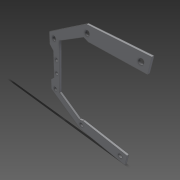
# Autodesk Inventor part: MuzzleHeadMount
Saved by Autodesk Inventor 2020 (Build 240168000, 168)
## iProperties
Created: 2021-07-18
Part Number: MuzzleHeadMount
Material: Generic
Document SubType Name: Sheet Metal
Designer: valer
Density: 1 g/cm^3
Sheet Metal Rule: Default
Appearance: Default
Author: valer
Autodesk Inventor part; units mm, degrees
ref_plane "YZ Plane" through (0, 0, 0) normal (1, 0, 0) x (0, 1, 0)
ref_plane "XZ Plane" through (0, 0, 0) normal (0, 1, 0) x (-1, 0, 0)
ref_plane "XY Plane" through (0, 0, 0) normal (0, 0, 1) x (1, 0, 0)
sketch "Sketch1" plane through (0, 0, 0) normal (0, 0, 1) x (1, 0, 0)
  circle A0 centre (0, 0) radius 3
  circle A1 centre (-6.2839, -68.2915) radius 2.875
  circle A2 centre (39.1052, -97.9753) radius 3
  circle A3 centre (99.0811, -103.4941) radius 3
  circle A4 centre (110.0198, 15.3837) radius 3
  circle A5 centre (50.0439, 20.9025) radius 3
  line L0 (-14.6913, -72.3521) -> (36.3914, -105.7594)
  line L1 (36.3914, -105.7594) -> (106.3144, -112.1934)
  line L2 (106.3144, -112.1934) -> (107.7805, -96.2608)
  line L3 (107.7805, -96.2608) -> (41.8191, -90.1913)
  line L4 (41.8191, -90.1913) -> (2.1235, -64.2309)
  line L5 (2.1235, -64.2309) -> (4.8244, -34.8788)
  line L6 (-178.2222, -18.0356) -> (255.5293, -57.9477) construction
  line L7 (-6.2839, -68.2915) -> (-3.142, -34.1457) construction
  line L8 (-6.2839, -68.2915) -> (39.1052, -97.9753) construction
  line L9 (39.1052, -97.9753) -> (99.0811, -103.4941) construction
  line L10 (-14.6913, -72.3521) -> (-11.1083, -33.4127)
  line L11 (4.8244, -34.8788) -> (-11.1083, -33.4127)
  line L12 (-7.5253, 5.5266) -> (48.7961, 29.0511)
  line L13 (48.7961, 29.0511) -> (118.7191, 22.617)
  line L14 (118.7191, 22.617) -> (117.2531, 6.6843)
  line L15 (117.2531, 6.6843) -> (51.2917, 12.7538)
  line L16 (51.2917, 12.7538) -> (7.5253, -5.5266)
  line L17 (7.5253, -5.5266) -> (4.8244, -34.8788)
  line L18 (-7.5253, 5.5266) -> (-11.1083, -33.4127)
  point P0 (0, 0)
  dimension "d0" = 8
  dimension "d1" = 8
  dimension "d2" = 8
  dimension "d3" = 8
  dimension "d4" = 8
  dimension "d5" = 8
  dimension "d6" = 8
  measures "d0" distance between parallel lines of L1 L9
  measures "d1" distance between parallel lines of L3 L9
  measures "d2" distance from line of L2 L9.end
  measures "d3" distance between parallel lines of L0 L8
  measures "d4" distance between parallel lines of L4 L8
  measures "d5" distance between parallel lines of L10 L7
  measures "d6" distance between parallel lines of L5 L7
extrude "Plate1" add sketch "Sketch1" along normal blind 3.048
sketch "Sketch2" plane through (0, 0, 3.048) normal (0, 0, 1) x (1, 0, 0)
  line L0 (-13.3312, -57.5708) -> (-6.8067, -52.1458)
  line L1 (-14.6913, -72.3521) -> (-7.5253, 5.5266) projected
  line L2 (7.5253, -5.5266) -> (2.1235, -64.2309) projected
  line L3 (-11.1083, -33.4127) -> (4.8244, -34.8788)
  line L4 (2.1235, -64.2309) -> (7.5253, -5.5266) projected
  line L5 (-6.8067, -52.1458) -> (-3.4604, -15.7791)
  line L6 (-3.4604, -15.7791) -> (-8.8854, -9.2546)
  point P0 (0, 0)
  point P1 (-5.1335, -33.9625)
  dimension "d8" = 45
  dimension "d9" = 45
  dimension "d10" = 6
  constraints: 8 end point, 3 midpoint, 3 point on line, 1 perpendicular
  measures "d8" angle of L1 L0
  measures "d9" angle of L1 L6
  measures "d10" distance between parallel lines of L1 L5
extrude "Cut1" cut sketch "Sketch2" against normal blind 3.048
sketch "Sketch3" plane through (0, 0, 3.048) normal (0, 0, 1) x (1, 0, 0)
  ellipse E0 centre (35.8905, -88.6417) end of major axis (36.1653, -85.6543) minor radius 2.9795 (33.3641, -87.0543) -> (38.664, -87.542) ccw projected
  ellipse E1 centre (45.1798, 12.3117) end of major axis (44.9049, 9.3243) minor radius 2.9795 (42.6535, 13.8991) -> (47.9534, 13.4114) ccw projected
  line L0 (41.8191, -90.1913) -> (107.7805, -96.2608) projected
  line L1 (41.8191, -90.1913) -> (35.3649, -91.8772)
  line L2 (35.3649, -91.8772) -> (1.6108, -69.8026)
  line L3 (7.5253, -5.5266) -> (2.1235, -64.2309) projected
  line L4 (1.6108, -69.8026) -> (2.1235, -64.2309)
  line L5 (2.1235, -64.2309) -> (41.8191, -90.1913) construction
  line L6 (-178.2222, -18.0356) -> (255.5293, -57.9477)
  line L7 (41.8191, -90.1913) -> (2.1235, -64.2309)
  line L8 (51.2917, 12.7538) -> (45.2535, 15.5893)
  line L9 (45.2535, 15.5893) -> (8.0379, 0.045)
  line L10 (8.0379, 0.045) -> (7.5253, -5.5266)
  line L11 (7.5253, -5.5266) -> (51.2917, 12.7538)
  point P0 (0, 0)
  constraints: 18 end point, 3 symmetric about line, 1 collinear, 1 parallel, 7 other
extrude "Cut2" cut sketch "Sketch3" against normal blind 3.048 contours L2 L4 L7 E0 | E0 L1 L2 | E0 L7 L1 | L11 L10 L9 L8
sketch "Sketch4" plane through (0, 0, 3.048) normal (0, 0, 1) x (1, 0, 0)
  line L0 (-3.4604, -15.7791) -> (-6.8067, -52.1458) projected
  line L1 (1.6108, -69.8026) -> (8.0379, 0.045) projected
  line L2 (-5.1335, -33.9625) -> (4.8244, -34.8788) construction
  line L3 (-0.1546, -34.4206) -> (-1.8277, -52.604) construction
  line L4 (-6.8067, -52.1458) -> (-3.4604, -15.7791) projected
  line L5 (-6.8067, -52.1458) -> (3.1512, -53.0621) construction
  circle A0 centre (-0.9912, -43.5123) radius 2.5
  circle A1 centre (0.682, -25.329) radius 2.5
  point P0 (0, 0)
  dimension "d15" = 5
  constraints: 6 end point, 5 midpoint, 2 centre point, 1 perpendicular, 1 point on line, 1 symmetric about line, 1 other
  measures "d15" diameter of A0
hole "Hole1" at (-0.9912, -43.5123, 3.048) at (0.682, -25.329, 3.048) direction (0, 0, -1) diameter 5 depth 3.048 tip angle 118
equation "\"d1\" = d0"
equation "\"d2\" = d0"
equation "\"d3\" = d0"
equation "\"d4\" = d0"
equation "\"d9\" = d8"
equation "\"d11\" = Thickness"
equation "\"d13\" = Thickness"
equation "\"d21\" = Thickness"
equation "\"d7\" = Thickness"
equation "\"BendRadius\" = Thickness"
equation "\"BendReliefWidth\" = Thickness"
equation "\"BendReliefDepth\" = 0.5 * Thickness"
equation "\"CornerReliefSize\" = 4 * Thickness"
equation "\"MinimumRemnant\" = 2 * Thickness"
equation "\"TransitionRadius\" = BendRadius"
equation "\"JacobiRadiusSize\" = BendRadius"
equation "\"GapSize\" = Thickness"
equation "\"Thickness\" = 3.048"
body "Solid1"
